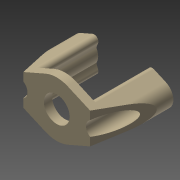
# Autodesk Inventor part: Encoder Mount
Saved by Autodesk Inventor 2014 SP1 (Build 180222100, 222)
## iProperties
Created: 2013-09-18
Part Number: Encoder Mount
Material: Generic
Document SubType Name: Modeling
Designer: grtstudent
Density: 1 g/cm^3
Mass: 3.6227 g
Surface Area: 32.9984 cm^2
Volume: 3.6227 cm^3
Appearance: Beige
Author: grtstudent
Autodesk Inventor part; units mm, degrees
ref_plane "YZ Plane" through (0, 0, 0) normal (1, 0, 0) x (0, 1, 0)
ref_plane "XZ Plane" through (0, 0, 0) normal (0, 1, 0) x (-1, 0, 0)
ref_plane "XY Plane" through (0, 0, 0) normal (0, 0, 1) x (1, 0, 0)
sketch "Sketch1" plane through (0, 0, 0) normal (0, 0, 1) x (1, 0, 0)
  arc A0 (9.5802, 4.2424) -> (-9.5802, 4.2424) centre (0, 0) ccw
  circle A1 centre (0, 0) radius 14.2875 construction
  line L0 (-14.2875, 0) -> (14.2875, 0) construction
  arc A2 (-16.1925, -4.3649) -> (-16.1925, 4.3649) centre (-14.2875, 0) ccw
  arc A3 (16.1925, 4.3649) -> (16.1925, -4.3649) centre (14.2875, 0) ccw
  line L1 (-16.1925, 4.3649) -> (-11.6668, 6.3401)
  line L2 (4.191, 9.6028) -> (11.6668, 6.3401)
  line L3 (16.1925, -4.3649) -> (11.6668, -6.3401)
  line L4 (-16.1925, -4.3649) -> (-11.6668, -6.3401)
  arc A4 (-11.6668, -6.3401) -> (-9.5802, -4.2424) centre (-11.0318, -4.8851) ccw
  arc A5 (-9.5802, 4.2424) -> (-11.6668, 6.3401) centre (-11.0318, 4.8851) ccw
  arc A6 (9.5802, 4.2424) -> (11.6668, 6.3401) centre (11.0318, 4.8851) ccw
  arc A7 (9.5802, -4.2424) -> (11.6668, -6.3401) centre (11.0318, -4.8851) ccw
  arc A8 (11.6668, 6.3401) -> (9.5802, 4.2424) centre (11.0318, 4.8851) ccw
  arc A9 (16.1925, -4.3649) -> (16.1925, 4.3649) centre (14.2875, 0) ccw
  arc A10 (11.6668, -6.3401) -> (9.5802, -4.2424) centre (11.0318, -4.8851) ccw
  arc A11 (10.4775, 0) -> (9.5802, 4.2424) centre (0, 0) ccw
  arc A12 (9.5802, -4.2424) -> (10.4775, 0) centre (0, 0) ccw
  line L5 (11.6668, -6.3401) -> (4.191, -9.6028)
  line L6 (11.6668, 6.3401) -> (16.1925, 4.3649)
  arc A13 (-11.6668, 6.3401) -> (-9.5802, 4.2424) centre (-11.0318, 4.8851) ccw
  arc A14 (-9.5802, -4.2424) -> (-11.6668, -6.3401) centre (-11.0318, -4.8851) ccw
  arc A15 (-16.1925, 4.3649) -> (-16.1925, -4.3649) centre (-14.2875, 0) ccw
  line L7 (-11.6668, 6.3401) -> (-4.191, 9.6028)
  line L8 (-11.6668, -6.3401) -> (-4.191, -9.6028)
  arc A16 (-9.5802, -4.2424) -> (9.5802, -4.2424) centre (0, 0) ccw
  arc A17 (-9.5802, 4.2424) -> (-9.5802, -4.2424) centre (0, 0) ccw
  circle A18 centre (-14.2875, 0) radius 3.175
  circle A19 centre (14.2875, 0) radius 3.175
  circle A20 centre (0, 0) radius 9.017
  dimension "d0" = 20.955
  dimension "d1" = 28.575
  dimension "d33" = 9.525
  dimension "d34" = 9.525
  dimension "d35" = 3.175
  dimension "d43" = 6.35
  dimension "d44" = 6.35
  dimension "d53" = 18.034
  constraints: 51 point on circle, 48 tangent, 21 centre point, 18 end point, 8 coincident, 3 equal radius, 1 horizontal, 1 midpoint, 1 point on line
  measures "d0" diameter of A0
  measures "d1" diameter of A1
  measures "d33" diameter of A2
  measures "d34" diameter of A3
  measures "d35" diameter of A5
  measures "d43" diameter of A18
  measures "d44" diameter of A19
  measures "d53" diameter of A20
extrude "Extrusion1" add sketch "Sketch1" against normal blind 3.175 contours A11 A3 A12 A16 A17 A2 A0 | A8 A6 A3 | A0 L2 A8 | A6 A3 A11 | A6 A3 A9 A10 A12 A11 | A3 A6 | L6 A3 A6 | A11 A12 A3 | A0 A5 L7 | A3 A10 A12 | A13 A2 A5 | A17 A2 A13 | A13 A2 L1 | L3 A10 A3 | A10 A3 | A3 A10 A7 | A7 L5 A16 | A13 A2 | A2 A17 A14 A15 A13 | A2 A17 | A17 A14 A2 | A2 A14 L4 | L8 A4 A16 | A14 A4 A2 | A2 A14 | A18 | A19 | A20
extrude "Extrusion2" add sketch "Sketch1" against normal blind 25.2793 contours A8 A6 A3 | A6 A3 A11 | A6 A3 A9 A10 A12 A11 | A3 A6 | L6 A3 A6 | A11 A12 A3 | A3 A10 A12 | A13 A2 A5 | A17 A2 A13 | A13 A2 L1 | L3 A10 A3 | A10 A3 | A3 A10 A7 | A13 A2 | A2 A17 A14 A15 A13 | A2 A17 | A17 A14 A2 | A2 A14 L4 | A14 A4 A2 | A2 A14 | A18 | A19
hole "Hole1" at (-14.2875, 0, 0) at (14.2875, 0, 0) direction (0, 0, -1) diameter 3.81 end through all clearance for "Flat Head Machine Screw (82)" size "#6" standard "Ansi Unified Screw Threads"
hole "Hole2" at (0, 0, 0) direction (0, 0, -1) diameter 9.8044 end through all clearance for "Flat Head Machine Screw (82)" size "3/8" standard "Ansi Unified Screw Threads"
sketch "Sketch4" plane through (0, 0, 0) normal (0, 1, 0) x (-1, 0, 0)
  line L0 (-12.7, 0) -> (-19.05, -18.9293)
  line L1 (12.7, 0) -> (19.05, -18.9293)
  line L2 (-12.7, 0) -> (12.7, 0) construction
  line L3 (-12.3825, -25.2793) -> (-16.1925, -25.2793) projected
  line L4 (-11.6668, -25.2793) -> (-9.5802, -25.2793) projected
  line L5 (-10.1917, -25.2794) -> (-9.5802, -25.2793) projected
  line L6 (-9.5802, -25.2793) -> (-11.6668, -25.2793) projected
  line L7 (-11.6668, -25.2793) -> (-16.1925, -25.2793) projected
  line L8 (-16.1925, -25.2793) -> (-16.1925, -25.2793) projected
  line L9 (-16.1925, -25.2793) -> (-11.6668, -25.2793) projected
  line L10 (16.1925, -25.2793) -> (12.3825, -25.2793) projected
  line L11 (11.6668, -25.2793) -> (9.5802, -25.2793) projected
  line L12 (9.5802, -25.2793) -> (10.1917, -25.2794) projected
  line L13 (9.5802, -25.2793) -> (11.6668, -25.2793) projected
  line L14 (11.6668, -25.2793) -> (16.1925, -25.2793) projected
  line L15 (16.1925, -25.2793) -> (16.1925, -25.2793) projected
  line L16 (16.1925, -25.2793) -> (11.6668, -25.2793) projected
  line L17 (-19.05, 0) -> (-19.05, -25.2793) projected
  line L18 (19.05, 0) -> (19.05, -25.2793) projected
  line L19 (-12.7, 0) -> (-19.05, 0)
  line L20 (-19.05, -18.9293) -> (-19.05, 0)
  line L21 (19.05, 0) -> (19.05, -12.6397)
  line L22 (19.05, 0) -> (12.7, 0)
  line L23 (10.1917, -25.2794) -> (9.5802, -25.2793) projected
  line L24 (10.1917, -25.2794) -> (10.1917, -25.2794) projected
  line L25 (-9.5802, -25.2793) -> (-10.1917, -25.2794) projected
  line L26 (-10.1917, -25.2794) -> (-10.1917, -25.2794) projected
  point P0 (0, 0)
  dimension "d36" = 12.7
  dimension "d37" = 12.7
  dimension "d38" = 0
  dimension "d39" = 6.35
  dimension "d40" = 6.35
  constraints: 14 end point, 2 point on line, 1 collinear, 1 horizontal, 1 midpoint
  measures "d36" distance of point (0, 0) L0.start
  measures "d37" distance of L1.start point (0, 0)
  measures "d38" distance from line of point (0, 0) L2
  measures "d39" distance from line of L3 L0.end
  measures "d40" distance of L18.end L1.end
extrude "Extrusion3" cut sketch "Sketch4" along normal through all both and the other way through all
extrude "Extrusion4" cut sketch "Sketch1" against normal blind 18.9293 contours A18 | A19
chamfer "Chamfer1" [suppressed]
chamfer "Chamfer2" [suppressed]
sketch "Sketch5" plane through (0, 0, 0) normal (0, 0, 1) x (1, 0, 0)
  line L0 (-11.0005, -7.2781) -> (-12.7, -5.0829) projected
  line L1 (-12.7, -5.8892) -> (-4.191, -9.6028) projected
  arc A0 (-4.191, -9.6028) -> (4.191, -9.6028) centre (0, 0) ccw projected
  line L2 (4.191, -9.6028) -> (12.7, -5.8892) projected
  line L3 (12.7, -5.0829) -> (11.0005, -7.2781) projected
  line L4 (12.7, -5.8892) -> (12.7, -2.7496) projected
  line L5 (11.0005, 7.2781) -> (12.7, 5.0829) projected
  line L6 (12.7, 5.8892) -> (4.191, 9.6028) projected
  arc A1 (4.191, 9.6028) -> (-4.191, 9.6028) centre (0, 0) ccw projected
  line L7 (-4.191, 9.6028) -> (-12.7, 5.8892) projected
  line L8 (-12.7, 5.0829) -> (-11.0005, 7.2781) projected
  line L9 (-12.7, -2.7496) -> (-12.7, -5.8892) projected
  circle A2 centre (0, 0) radius 9.0488
  point P0 (-12.7, 5.8892)
  dimension "d54" = 18.0975
  constraints: 1 centre point, 1 coincident, 4 other
  measures "d54" diameter of A2
extrude "Extrusion5" [suppressed]
equation "\"d37\" = d36"
equation "\"d39\" = d40"
body "Solid1"
